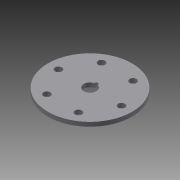
# Autodesk Inventor part: Fitting piece for Sprocket
Saved by Autodesk Inventor 2013 (Build 170138000, 138)
## iProperties
Created: 2013-01-31
Part Number: Fitting piece for Sprocket
Material: Generic
Document SubType Name: Sheet Metal
Designer: aslane
Density: 1 g/cm^3
Sheet Metal Rule: Default
Author: aslane
Autodesk Inventor part; units mm, degrees
ref_plane "YZ Plane" through (0, 0, 0) normal (1, 0, 0) x (0, 1, 0)
ref_plane "XZ Plane" through (0, 0, 0) normal (0, 1, 0) x (-1, 0, 0)
ref_plane "XY Plane" through (0, 0, 0) normal (0, 0, 1) x (1, 0, 0)
sketch "Sketch1" plane through (0, 0, 0) normal (0, 1, 0) x (-1, 0, 0)
  circle A0 centre (0, 0) radius 31.75
  line L0 (0, 0) -> (23.8252, 0)
  circle A1 centre (23.8252, 0) radius 2.6162
  circle A2 centre (11.9126, 20.6332) radius 2.6162
  circle A3 centre (-11.9126, 20.6332) radius 2.6162
  circle A4 centre (-23.8252, 0) radius 2.6162
  circle A5 centre (-11.9126, -20.6332) radius 2.6162
  circle A6 centre (11.9126, -20.6332) radius 2.6162
  dimension "d0" = 63.5
  dimension "d1" = 23.8252
  dimension "d2" = 5.2324
  dimension "d5" = 360
  measures "d0" diameter of A0
  measures "d1" distance of L0.start L0.end
  measures "d2" diameter of A1
extrude "Plate1" add sketch "Sketch1" along normal blind 3.175
sketch "Sketch2" plane through (0, 3.175, 0) normal (0, 1, 0) x (1, 0, 0)
  circle A0 centre (0, 0) radius 31.75 projected
  circle A1 centre (0, 0) radius 4.7625
  line L0 (0, 4.7625) -> (0, 4.2799)
  line L1 (1.1906, 4.2799) -> (1.1906, 4.6113)
  line L2 (-1.1906, 4.2799) -> (-1.1906, 4.6113)
  line L3 (0, 4.7625) -> (0, 5.9531)
  line L4 (0, 5.9531) -> (1.1906, 5.9531)
  line L5 (1.1906, 5.9531) -> (1.1906, 4.6113)
  line L6 (0, 5.9531) -> (-1.1906, 5.9531)
  line L7 (-1.1906, 5.9531) -> (-1.1906, 4.6113)
  dimension "d8" = 9.525
  dimension "d9" = 0.4826
  dimension "d10" = 1.1906
  dimension "d11" = 2.3813
  dimension "d12" = 1.1906
  constraints: 16 end point, 3 perpendicular, 3 point on circle, 2 parallel, 1 centre point, 1 coincident, 1 vertical
  measures "d8" diameter of A1
  measures "d9" distance of L0.start L0.end
  measures "d10" distance of L0.end L1.start
  measures "d11" distance of L1.start L2.start
  measures "d12" distance of L0.start L3.end
extrude "Cut1" cut sketch "Sketch2" against normal blind 3.175 contours A1 | A1 L3 L4 L5 | L7 L6 L3 A1
equation "\"d13\" = Thickness"
equation "\"BendRadius\" = Thickness"
equation "\"BendReliefWidth\" = Thickness"
equation "\"BendReliefDepth\" = 0.5 * Thickness"
equation "\"CornerReliefSize\" = 4 * Thickness"
equation "\"MinimumRemnant\" = 2 * Thickness"
equation "\"TransitionRadius\" = BendRadius"
equation "\"JacobiRadiusSize\" = BendRadius"
equation "\"GapSize\" = Thickness"
equation "\"d7\" = BendRadius"
equation "\"Thickness\" = 3.175"
body "Solid1"
